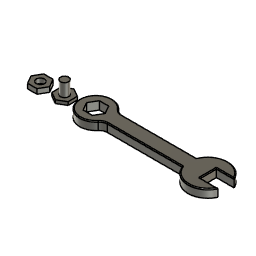
Tuerca v1 (Autodesk Fusion 360 design; units mm, degrees)
Autodesk Fusion 360 part; units mm, degrees
sketch "Boceto1" plane through (0, 0, 0) normal (0, 0, 1) x (1, 0, 0)
  line L0 (11.547, 0) -> (5.7735, 10)
  line L1 (5.7735, 10) -> (-5.7735, 10)
  line L2 (-5.7735, 10) -> (-11.547, 0)
  line L3 (-11.547, 0) -> (-5.7735, -10)
  line L4 (-5.7735, -10) -> (5.7735, -10)
  line L5 (5.7735, -10) -> (11.547, 0)
  circle A0 centre (0, 0) radius 5
  dimension "d1" = 10
  dimension "d2" = 10
  constraint coincident A0.centre origin
  constraint horizontal L1
  measures "d1" distance of A0.centre L5
  measures "d2" diameter of A0
extrude "Extruir1" add sketch "Boceto1" along normal mid plane 6 makes body 1
cylinder "CilindroPrimitivo1" add diameter 10 height 20 placed x (1, 0, 0) y (0, 1, 0) z (0, 0, 1) at (30, 0, 0) separate body makes body 2
sketch "Boceto3" plane through (0, 0, 0) normal (0, 0, -1) x (1, 0, 0)
  circle A0 centre (30, 0) radius 5
  line L0 (40.0553, 5.6766) -> (30.1116, 11.5465)
  line L1 (30.1116, 11.5465) -> (20.0563, 5.8699)
  line L2 (20.0563, 5.8699) -> (19.9447, -5.6766)
  line L3 (19.9447, -5.6766) -> (29.8884, -11.5465)
  line L4 (29.8884, -11.5465) -> (39.9437, -5.8699)
  line L5 (39.9437, -5.8699) -> (40.0553, 5.6766)
  point P0 (30, 0)
  dimension "d7" = 10
  constraint coincident P0 A0.centre
  measures "d7" distance of P0 L5
extrude "Extruir2" add sketch "Boceto3" against normal blind 4 bodies 2
sketch "Boceto4" plane through (0, 0, 0) normal (0, 0, 1) x (1, 0, 0)
  line L0 (74.3139, 8.7275) -> (68.4534, -1.2218)
  line L1 (68.4534, -1.2218) -> (74.1395, -11.2718)
  line L2 (74.1395, -11.2718) -> (85.6861, -11.3724)
  line L3 (85.6861, -11.3724) -> (91.5466, -1.4232)
  line L4 (91.5466, -1.4232) -> (85.8605, 8.6268)
  line L5 (85.8605, 8.6268) -> (74.3139, 8.7275)
  line L6 (241, -11.3225) -> (219, -11.3225)
  line L7 (219, -11.3225) -> (219, 8.6775)
  line L8 (219, 8.6775) -> (241, 8.6775)
  line L9 (241, -11.3225) -> (219, 8.6775) construction
  line L10 (219, -11.3225) -> (241, 8.6775) construction
  line L11 (97.8606, 7.6775) -> (195.7103, 7.6775)
  line L12 (97.8606, -10.3225) -> (195.7103, -10.3225)
  arc A0 (241, 8.6775) -> (195.7103, 7.6775) centre (218.5649, -1.3225) ccw
  arc A1 (195.7103, -10.3225) -> (241, -11.3225) centre (218.5649, -1.3225) ccw
  arc A2 (97.8606, 7.6775) -> (97.8606, -10.3225) centre (80, -1.3225) ccw
  point P0 (80, -1.3225)
  point P1 (230, -1.3225)
  dimension "d10" = 150
  dimension "d11" = 10
  dimension "d12" = 40
  dimension "d13" = 22
  dimension "d14" = 20
  constraint coincident P0 A2.centre
  constraint horizontal L6
  constraint perpendicular L6 L7
  constraint parallel L6 L8
  constraint coincident L9 P1
  constraint coincident L10 P1
  constraint concentric A0 A1
  measures "d10" distance of P0 P1
  measures "d11" distance of P0 L5
  measures "d12" diameter of A2
  measures "d13" distance of L7.end L8.end
  measures "d14" distance of L6.start L8.end
extrude "Extruir3" add sketch "Boceto4" along normal blind 10 separate body makes body 3
fillet "Empalme1" radius 10 2 edges at (97.8606, -10.3225, 5) (97.8606, 7.6775, 5) on bodies 3
fillet "Empalme2" radius 1 10 edges at (149.4633, 7.6775, 10) (98.9346, 8.6405, 10) (60, -1.3225, 10) (98.9346, -11.2855, 10) (149.4633, -10.3225, 10) (218.0227, 23.2344, 10) (219, -1.3225, 10) (230, -11.3225, 10) (230, 8.6775, 10) (218.0227, -25.8794, 10) on bodies 3
move_body "Desplazar1" bodies 3 to x (1, 0, 0) y (0, 1, 0) z (0, 0, 1) at (-10, 0, 0)
